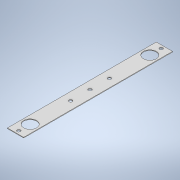
# Autodesk Inventor part: chassisPart1
Saved by Autodesk Inventor 2020.3 (Build 243373000, 373)
## iProperties
Created: 2022-07-01
Part Number: chassisPart1
Material: Generic
Document SubType Name: Sheet Metal
Designer: 0x6f736f646f
Density: 1 g/cm^3
Sheet Metal Rule: Default_mm
Appearance: Default
Author: 0x6f736f646f
Autodesk Inventor part; units mm, degrees
ref_plane "YZ Plane" through (0, 0, 0) normal (1, 0, 0) x (0, 1, 0)
ref_plane "XZ Plane" through (0, 0, 0) normal (0, 1, 0) x (-1, 0, 0)
ref_plane "XY Plane" through (0, 0, 0) normal (0, 0, 1) x (1, 0, 0)
sketch "Sketch1" plane through (0, 0, 0) normal (0, 1, 0) x (-1, 0, 0)
  line L0 (0, 0) -> (50, 0)
  line L1 (50, 0) -> (50, 460)
  line L2 (50, 460) -> (0, 460)
  line L3 (0, 460) -> (0, 0)
  circle A0 centre (25, 415) radius 20
  circle A1 centre (25, 45) radius 20
  circle A2 centre (25, 450) radius 5
  circle A3 centre (25, 10) radius 5
  line L4 (50, 280) -> (0, 280)
  line L5 (0, 280) -> (0, 180)
  line L6 (0, 180) -> (50, 180)
  line L7 (50, 180) -> (50, 280)
  circle A4 centre (25, 170) radius 5
  circle A5 centre (25, 290) radius 5
  circle A6 centre (25, 230) radius 5
  dimension "d0" = 50
  dimension "d1" = 460
  dimension "d2" = 45
  dimension "d3" = 40
  dimension "d4" = 45
  dimension "d5" = 10
  dimension "d6" = 10
  dimension "d7" = 10
  dimension "d8" = 10
  dimension "d9" = 25
  dimension "d10" = 25
  dimension "d11" = 25
  dimension "d12" = 25
  dimension "d15" = 50
  dimension "d16" = 100
  dimension "d17" = 180
  dimension "d18" = 10
  dimension "d20" = 10
  dimension "d21" = 10
  dimension "d22" = 25
  dimension "d23" = 25
  dimension "d24" = 10
  dimension "d27" = 10
  dimension "d28" = 25
  dimension "d29" = 50
  measures "d0" distance of L2.end L1.end
  measures "d1" distance of L1.end L0.end
  measures "d2" distance from line of L0 A1.centre
  measures "d3" diameter of A1
  measures "d4" distance from line of L2 A0.centre
  measures "d5" diameter of A3
  measures "d6" diameter of A2
  measures "d7" distance from line of L0 A3.centre
  measures "d8" distance from line of A2.centre L2
  measures "d9" distance from line of L3 A3.centre
  measures "d10" distance from line of L3 A1.centre
  measures "d11" distance from line of L3 A2.centre
  measures "d12" distance from line of L3 A0.centre
  measures "d15" distance of L6.end L5.end
  measures "d16" distance of L5.end L4.end
  measures "d17" distance between parallel lines of L6 L0
  measures "d18" diameter of A4
  measures "d20" diameter of A5
  measures "d21" distance from line of L4 A5.centre
  measures "d22" distance from line of A5.centre L1
  measures "d23" distance from line of A4.centre L1
  measures "d24" distance from line of L6 A4.centre
  measures "d27" diameter of A6
  measures "d28" distance from line of L5 A6.centre
  measures "d29" distance from line of L6 A6.centre
extrude "Plate3" add sketch "Sketch1" along normal blind 2
equation "\"d30\" = Thickness"
equation "\"BendRadius\" = Thickness"
equation "\"BendReliefWidth\" = Thickness"
equation "\"BendReliefDepth\" = 0.5 * Thickness"
equation "\"CornerReliefSize\" = 4 * Thickness"
equation "\"MinimumRemnant\" = 2 * Thickness"
equation "\"TransitionRadius\" = BendRadius"
equation "\"JacobiRadiusSize\" = BendRadius"
equation "\"GapSize\" = Thickness"
equation "\"Thickness\" = 2"
body "Solid3"
